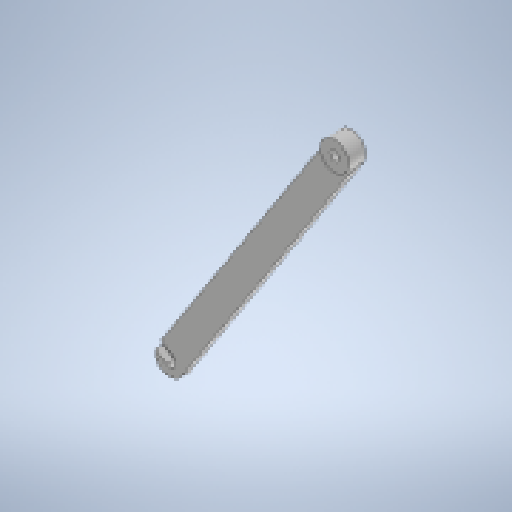
# Autodesk Inventor part: TheHandle
Saved by Autodesk Inventor 2025.1 (Build 291241000, 241)
## iProperties
Created: 2026-05-10
Part Number: TheHandle
Material: Generic
Document SubType Name: Modeling
Designer: User
Density: 1 g/cm^3
Appearance: Default
Author: User
## iProperties of the stored document TheHandle_Right_3DPrint.ipt
Created: 2026-05-12
Part Number: TheHandle_Right_3DPrint
Material: Generic
Document SubType Name: Modeling
Designer: User
Density: 1 g/cm^3
Appearance: Default
Author: User
Autodesk Inventor part; units mm, degrees
ref_plane "YZ Plane" through (0, 0, 0) normal (1, 0, 0) x (0, 1, 0)
ref_plane "XZ Plane" through (0, 0, 0) normal (0, 1, 0) x (-1, 0, 0)
ref_plane "XY Plane" through (0, 0, 0) normal (0, 0, 1) x (1, 0, 0)
sketch "Sketch1" plane through (0, 0, 0) normal (0, 0, 1) x (1, 0, 0)
  circle A0 centre (33.7394, 8.5) radius 2.5 projected
  circle A1 centre (-57.3324, -132.0207) radius 2.5 projected
  circle A2 centre (33.7394, 8.5) radius 7.5
  line L0 (40.0332, 4.421) -> (-51.0386, -136.0997)
  arc A3 (-64.7058, -130.6488) -> (-58.937, -134.5557) centre (33.7394, 8.5) ccw
  line L1 (27.4456, 12.579) -> (-61.9015, -125.2806)
  arc A4 (-64.7058, -130.6488) -> (-51.0386, -136.0997) centre (-57.3324, -132.0207) ccw
  arc A5 (-58.991, -134.5207) -> (-55.7273, -129.486) centre (-57.3324, -132.0207) ccw
  arc A6 (-61.9015, -125.2806) -> (-55.6742, -129.5204) centre (33.7394, 8.5) ccw
  point P0 (0, 0)
  dimension "d1" = 15
  constraints: 14 point on circle, 5 centre point, 4 coincident, 4 end point, 3 tangent
  measures "d1" diameter of A2
extrude "Extrusion1" add sketch "Sketch1" along normal blind 4 contours A2 | A2 L0 A4 A3 A5 A6 L1
sketch "Sketch2" plane through (0, 0, 4) normal (0, 0, 1) x (1, 0, 0)
  circle A0 centre (33.7394, 8.5) radius 2.5
  circle A1 centre (33.7394, 8.5) radius 7.5
  point P0 (0, 0)
  constraints: 2 centre point, 1 coincident, 2 other
ref_plane "Work Plane1" through (-39.4645, -13.5002, 8.8802) normal (0, 0, -1) x (-0.0000023, 1, 0)
extrude "Extrusion2" add sketch "Sketch2" along normal up to surface (4.8802 mm away)
sketch "Sketch3" plane through (0, 0, 0) normal (0, 0, -1) x (-1, 0, 0)
  arc A0 (58.991, -134.5207) -> (64.7058, -130.6488) centre (-33.7394, 8.5) ccw projected
  arc A1 (51.0386, -136.0997) -> (64.7058, -130.6488) centre (57.3324, -132.0207) ccw projected
  line L0 (51.0386, -136.0997) -> (-40.0332, 4.421) projected
  line L1 (-43.3899, 2.2455) -> (47.6819, -138.2752)
  arc A2 (47.6819, -138.2752) -> (66.1549, -124.6441) centre (57.3324, -132.0207) ccw
  arc A3 (56.8149, -131.1644) -> (66.1549, -124.6441) centre (-33.7394, 8.5) ccw
  arc A4 (58.991, -134.5207) -> (64.7058, -130.6488) centre (-33.7394, 8.5) ccw projected
  line L2 (58.991, -134.5207) -> (64.7058, -130.6488)
  arc A5 (55.7273, -129.486) -> (58.991, -134.5207) centre (57.3324, -132.0207) ccw projected
  line L3 (58.991, -134.5207) -> (68.2061, -128.2773)
  line L4 (-31.6873, -15.8111) -> (-20.0095, 1.1054)
  line L5 (-26.8752, -15.8813) -> (-17.6559, -2.5262)
  line L6 (-27.4456, 12.579) -> (61.9015, -125.2806) projected
  point P0 (0, 0)
  point P1 (64.7058, -130.6488)
  dimension "d9" = 4
  constraints: 10 end point, 5 point on circle, 2 centre point, 1 point on line, 8 other
  measures "d9" distance between parallel lines of L0 L1
extrude "Extrusion3" add sketch "Sketch3" along normal mid plane 8 contours L3 A2 L1 L4 L0 A1 | L0 L4 L6 L5
sketch "Sketch4" plane through (0, 0, 0) normal (0, 0, -1) x (-1, 0, 0)
  line L0 (-29.2288, -12.2498) -> (-40.0332, 4.421) projected
  line L1 (-31.6873, -15.8111) -> (-29.2288, -12.2498) projected
  arc A0 (-27.4456, 12.579) -> (-40.0332, 4.421) centre (-33.7394, 8.5) ccw projected
  line L2 (47.6819, -138.2752) -> (-31.6873, -15.8111) projected
  line L3 (-31.6873, -15.8111) -> (-46.724, 20.086)
  point P0 (0, 0)
  point P1 (-40.657, 5.6023)
  constraints: 2 end point, 1 tangent
extrude "Extrusion4" add sketch "Sketch4" against normal blind 4
sketch "Sketch5" plane through (33.7394, 8.5, 8.8802) normal (0, 0, 1) x (1, 0, 0)
  line L0 (-7.5, 0) -> (-7.5005, 100.4366)
  line L1 (7.4995, 100.4366) -> (7.5, 0)
  arc A0 (7.4995, 100.4366) -> (-7.5005, 100.4366) centre (-0.0005, 100.4366) ccw
  circle A1 centre (-0.0005, 100.4366) radius 2.5
  circle A2 centre (0, 0) radius 7.5 projected
  circle A3 centre (0, 0) radius 2.5 projected
  point P0 (-33.7394, -8.5)
  constraints: 4 end point, 2 centre point, 2 point on circle, 10 other
extrude "Extrusion5" add sketch "Sketch5" against normal up to surface (8.8802 mm away) contours L0 A0 L1 A2
chamfer "Chamfer1" distance 4.5 angle 45 2 edges at (32.2616, 1.147, 4) (26.2394, 9.6089, 4)
chamfer "Chamfer2" distance 4.5 angle 45 1 edges at (26.2394, 10.7178, 4.25)
sketch "Sketch6" plane through (0, 0, 0) normal (0, 0, -1) x (-1, 0, 0)
  line L0 (-41.2389, 108.9366) -> (-41.2394, 8.5) projected
  line L1 (-26.2394, 15.2178) -> (-26.2389, 108.9366) projected
  arc A0 (-26.2389, 108.9366) -> (-41.2389, 108.9366) centre (-33.7389, 108.9366) ccw projected
  line L2 (-22.2394, 15.2178) -> (-22.2389, 108.9365)
  arc A1 (-22.2389, 108.9365) -> (-45.2389, 108.9366) centre (-33.7389, 108.9366) ccw
  line L3 (-45.2389, 108.9366) -> (-45.2394, 8.5001)
  arc A2 (-41.2394, 8.5) -> (-40.657, 5.6023) centre (-33.7394, 8.5) ccw projected
  line L4 (-26.2394, 15.2178) -> (-23.792, 6.9416) projected
  arc A3 (-25.5098, 2.819) -> (-41.969, 14.181) centre (-33.7394, 8.5) ccw
  arc A4 (-22.218, 0.5466) -> (-45.2608, 16.4534) centre (-33.7394, 8.5) ccw
  line L5 (-41.2393, 20.3216) -> (-45.2393, 24.3216)
  line L6 (-41.2393, 20.3216) -> (-35.5825, 20.3216) construction
  line L7 (-26.2389, 108.9366) -> (-26.2394, 8.5) projected
  line L8 (-26.2393, 20.3216) -> (-22.2393, 24.3216)
  line L9 (-26.2393, 20.3216) -> (-20.5825, 20.3216) construction
  point P0 (0, 0)
  point P1 (-26.2393, 20.3216)
  dimension "d22" = 4
  dimension "d23" = 4
  dimension "d24" = 135
  dimension "d25" = 45
  constraints: 12 end point, 8 point on circle, 4 point on line, 3 centre point, 2 equal length, 2 horizontal, 6 other
  measures "d22" distance between parallel lines of L1 L2
  measures "d23" radial gap between concentric circles of A3 A4
  measures "d24" angle of L6 L5
  measures "d25" angle of L9 L8
extrude "Extrusion6" add sketch "Sketch6" along normal mid plane 10 contours L0 L5 L3 A1 L2 L8 L1 A0
chamfer "Chamfer3" distance 3.88 angle 45 3 edges at (26.2391, 64.6291, 5) (33.7389, 116.4366, 5) (41.2391, 64.6291, 5)
sketch "Sketch7" plane through (0, 0, 0) normal (0, 0, -1) x (-1, 0, 0)
  line L0 (-20.0095, 1.1054) -> (-31.6873, -15.8111) projected
  circle A0 centre (-33.7394, 8.5) radius 2.5
  line L1 (-23.792, 6.9416) -> (-20.0095, 1.1054) projected
  circle A1 centre (-33.7394, 8.5) radius 15.5945
  line L2 (-26.8752, -15.8813) -> (-17.6559, -2.5262) projected
  circle A2 centre (-33.7394, 8.5) radius 19.5001
  line L3 (-26.2393, 20.3216) -> (-26.2389, 108.9366) projected
  line L4 (-26.2394, 15.2178) -> (-26.2393, 20.3216) projected
  line L5 (-17.6559, -2.5262) -> (-20.0095, 1.1054) projected
  point P0 (0, 0)
  point P1 (-26.2393, 26.5001)
  point P2 (-26.2393, 22.1725)
  constraints: 2 centre point, 2 coincident, 5 other
extrude "Extrusion7" add sketch "Sketch7" along normal mid plane 8 contours A1 L3 A2 L5
sketch "Sketch8" plane through (0, 0, 0) normal (0, 0, -1) x (-1, 0, 0)
  line L0 (-26.2394, 15.2178) -> (-26.2393, 20.3216) projected
  line L1 (-26.2394, 15.2178) -> (-23.792, 6.9416) projected
  line L2 (-23.792, 6.9416) -> (-20.0095, 1.1054) projected
  arc A0 (-20.0095, 1.1054) -> (-25.0869, 21.474) centre (-33.7394, 8.5) ccw projected
  line L3 (-26.2393, 20.3216) -> (-22.2393, 24.3216) projected
  point P0 (0, 0)
extrude "Extrusion8" add sketch "Sketch8" against normal up to surface (4 mm away)
chamfer "Chamfer4" distance 1 angle 45 1 edges at (24.2393, 22.3216, -5)
sketch "Sketch9" plane through (0, 0, -5) normal (0, 0, -1) x (-1, 0, 0)
  arc A0 (-20.0095, 1.1054) -> (-25.0869, 21.474) centre (-33.7394, 8.5) ccw projected
  line L0 (-26.2389, 108.9366) -> (-26.2393, 21.7358) projected
  line L1 (-26.2393, 20.3216) -> (-25.0869, 21.474) projected
  line L2 (-26.2393, 21.7358) -> (-26.2393, 20.3216) projected
  circle A1 centre (-33.7394, 8.5) radius 15.5945
  point P0 (0, 0)
  point P1 (-25.0869, 21.474)
  point P2 (-26.2393, 22.1725)
  constraints: 1 centre point, 1 coincident, 1 concentric
extrude "Extrusion9" cut sketch "Sketch9" against normal up to surface (5 mm away) contours A1 L1 L2 L0
sketch "Sketch10" plane through (0, 0, -4) normal (0, 0, -1) x (-1, 0, 0)
  arc A0 (51.0386, -136.0997) -> (64.7058, -130.6488) centre (57.3324, -132.0207) ccw projected
  arc A1 (47.6819, -138.2752) -> (68.2061, -128.2773) centre (57.3324, -132.0207) ccw projected
  line L0 (68.2061, -128.2773) -> (64.7058, -130.6488) projected
  arc A2 (55.7273, -129.486) -> (58.991, -134.5207) centre (57.3324, -132.0207) ccw projected
  line L1 (57.3324, -132.0207) -> (61.4714, -138.2752)
  line L2 (61.4714, -138.2752) -> (68.7414, -133.4641)
  point P0 (0, 0)
  constraints: 4 end point, 2 point on circle, 1 perpendicular, 1 tangent
extrude "Extrusion10" cut sketch "Sketch10" against normal up to surface (4 mm away)
sketch "Sketch11" plane through (0, 0, -4) normal (0, 0, -1) x (-1, 0, 0)
  line L0 (51.0386, -136.0997) -> (-26.8752, -15.8813) projected
  arc A0 (51.0386, -136.0997) -> (61.4714, -138.2752) centre (57.3324, -132.0207) ccw projected
  line L1 (68.7414, -133.4641) -> (61.4714, -138.2752) projected
  line L2 (69.0174, -133.8811) -> (61.7473, -138.6921)
  arc A1 (50.619, -136.3716) -> (61.7473, -138.6921) centre (57.3324, -132.0207) ccw
  line L3 (50.619, -136.3716) -> (-27.2948, -16.1532)
  circle A2 centre (57.3324, -132.0207) radius 8
  arc A3 (47.6819, -138.2752) -> (68.7414, -133.4641) centre (57.3324, -132.0207) ccw projected
  point P0 (0, 0)
  point P1 (68.6367, -134.133)
  point P2 (49.5245, -133.7635)
  point P3 (50.619, -136.3716)
  dimension "d42" = 0.5
  constraints: 4 end point, 2 centre point, 2 point on circle, 1 coincident, 1 tangent, 2 other
  measures "d42" radial gap between concentric circles of A0 A1
extrude "Extrusion11" cut sketch "Sketch11" against normal up to surface (4 mm away) contours A0 L1 A2 A1 L0 | L1 A3 L2 A2
sketch "Sketch12" plane through (0, 0, 0) normal (0, 0, -1) x (-1, 0, 0)
  line L0 (16.2758, -60.4779) -> (26.6623, -76.4412) construction
  line L1 (26.6623, -76.4412) -> (17.781, -82.2197) construction
  line L2 (17.781, -82.2197) -> (7.3945, -66.2565) construction
  line L3 (7.3945, -66.2565) -> (16.2758, -60.4779) construction
  line L4 (13.3339, -75.3744) -> (11.5695, -72.6626)
  line L5 (11.5695, -72.6626) -> (13.2227, -68.0751)
  line L6 (13.2227, -68.0751) -> (12.6985, -67.2695)
  line L7 (12.6985, -67.2695) -> (9.4399, -69.3896)
  line L8 (9.4399, -69.3896) -> (7.9984, -67.1741)
  line L9 (7.9984, -67.1741) -> (16.8749, -61.3986)
  line L10 (16.8749, -61.3986) -> (19.1963, -64.9665)
  spline S0 degree 2 poles (19.1963, -64.9665) (19.6784, -65.7074) (20.2028, -66.9225) (20.2192, -67.5772) knots 0 0 0 1 2 2 2
  spline S1 degree 2 poles (20.2192, -67.5772) (20.226, -68.2486) (19.6488, -69.4228) (18.9294, -69.8908) knots 0 0 0 1 2 2 2
  spline S2 degree 2 poles (18.9294, -69.8908) (17.9152, -70.5507) (16.0429, -70.4584) (15.1681, -69.9321) knots 0 0 0 1 2 2 2
  line L11 (15.1681, -69.9321) -> (13.3339, -75.3744)
  spline S3 degree 2 poles (17.1606, -67.7859) (17.4987, -67.5659) (17.8121, -66.9934) (17.7497, -66.6142) knots 0 0 0 1 2 2 2
  spline S4 degree 2 poles (17.7497, -66.6142) (17.7003, -66.3494) (17.4183, -65.8059) (17.1703, -65.4247) knots 0 0 0 1 2 2 2
  line L12 (17.1703, -65.4247) -> (16.6835, -64.6766)
  line L13 (16.6835, -64.6766) -> (14.2954, -66.2305)
  line L14 (14.2954, -66.2305) -> (14.7119, -66.8707)
  spline S5 degree 2 poles (14.7119, -66.8707) (15.0115, -67.331) (15.5525, -67.9107) (15.8774, -68.0167) knots 0 0 0 1 2 2 2
  spline S6 degree 2 poles (15.8774, -68.0167) (16.1904, -68.1202) (16.7865, -68.0292) (17.1606, -67.7859) knots 0 0 0 1 2 2 2
  line L15 (24.8165, -77.3022) -> (22.3921, -73.5761)
  line L16 (22.3921, -73.5761) -> (20.7161, -74.6666)
  line L17 (20.7161, -74.6666) -> (22.9486, -78.0978)
  line L18 (22.9486, -78.0978) -> (21.2582, -79.1977)
  line L19 (21.2582, -79.1977) -> (19.0257, -75.7665)
  line L20 (19.0257, -75.7665) -> (15.206, -78.2517)
  line L21 (15.206, -78.2517) -> (13.7645, -76.0362)
  line L22 (13.7645, -76.0362) -> (22.641, -70.2607)
  line L23 (22.641, -70.2607) -> (26.5069, -76.2024)
  line L24 (26.5069, -76.2024) -> (24.8165, -77.3022)
  point P0 (0, 0)
  constraints: 2 other
emboss "Emboss1" sketch "Sketch12" operation cut depth 0.5 direction (0, 0, 1)
body "Solid1"
